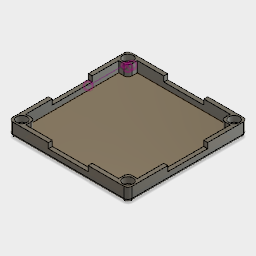
stage0 v2 (Autodesk Fusion 360 design; units mm, degrees)
Autodesk Fusion 360 part; units mm, degrees
sketch "Sketch1" plane through (0, 0, 0) normal (0, 1, 0) x (1, 0, 0)
  line L0 (0, 0) -> (90, 0)
  line L1 (90, 0) -> (90, 90)
  line L2 (90, 90) -> (0, 90)
  line L3 (0, 90) -> (0, 0)
  dimension "d1" = 90
  dimension "d2" = 90
  measures "d1" distance of L0.start L2.end
  measures "d2" distance of L0.start L0.end
extrude "Extrude1" add sketch "Sketch1" along normal blind 11
sketch "Sketch2" plane through (0, 11, 0) normal (0, 1, 0) x (-1, 0, 0)
  line L0 (0, -90) -> (0, 0)
  line L1 (0, 0) -> (-90, 0)
  line L2 (-90, 0) -> (-90, -90)
  line L3 (-90, -90) -> (0, -90)
  circle A0 centre (-5, -85) radius 3.875
  circle A1 centre (-5, -5) radius 3.875
  circle A2 centre (-85, -5) radius 3.875
  circle A3 centre (-85, -85) radius 3.875
  dimension "d5" = 7.75
  dimension "d6" = 7.75
  dimension "d7" = 7.75
  dimension "d8" = 7.75
  measures "d5" diameter of A0
  measures "d6" diameter of A1
  measures "d7" diameter of A2
  measures "d8" diameter of A3
extrude "Extrude2" cut sketch "Sketch2" against normal blind 4.5 contours A0 | A1 | A2 | A3
sketch "Sketch3" plane through (0, 11, 0) normal (0, 1, 0) x (-1, 0, 0)
  circle A0 centre (-85, -85) radius 3.875
  circle A1 centre (-5, -5) radius 3.875
  circle A2 centre (-5, -85) radius 3.875
  circle A3 centre (-85, -5) radius 3.875
  line L0 (0, -90) -> (0, 0)
  line L1 (0, 0) -> (-90, 0)
  line L2 (-90, 0) -> (-90, -90)
  line L3 (-90, -90) -> (0, -90)
  line L4 (-90, -80) -> (-90, -10)
  line L5 (0, -10) -> (0, -80)
  line L6 (-10, -90) -> (-80, -90)
  line L7 (-80, 0) -> (-10, 0)
  line L8 (-10, 0) -> (-10, -7)
  line L9 (-10, -83) -> (-10, -90)
  line L10 (-90, -10) -> (-83, -10)
  line L11 (-7, -10) -> (0, -10)
  line L12 (-80, -90) -> (-80, -83)
  line L13 (-80, -7) -> (-80, 0)
  line L14 (0, -80) -> (-7, -80)
  line L15 (-83, -80) -> (-90, -80)
  line L16 (0, -10) -> (-3, -10)
  line L17 (-3, -10) -> (-3, -30)
  line L18 (-3, -30) -> (0, -30)
  line L19 (0, -30) -> (0, -10)
  line L20 (0, -80) -> (-3, -80)
  line L21 (-3, -80) -> (-3, -60)
  line L22 (-3, -60) -> (0, -60)
  line L23 (0, -60) -> (0, -80)
  line L24 (-10, -90) -> (-30, -90)
  line L25 (-30, -90) -> (-30, -87)
  line L26 (-30, -87) -> (-10, -87)
  line L27 (-10, -87) -> (-10, -90)
  line L28 (-80, -90) -> (-60, -90)
  line L29 (-60, -90) -> (-60, -87)
  line L30 (-60, -87) -> (-80, -87)
  line L31 (-80, -87) -> (-80, -90)
  line L32 (-90, -80) -> (-87, -80)
  line L33 (-87, -80) -> (-87, -60)
  line L34 (-87, -60) -> (-90, -60)
  line L35 (-90, -60) -> (-90, -80)
  line L36 (-90, -10) -> (-87, -10)
  line L37 (-87, -10) -> (-87, -30)
  line L38 (-87, -30) -> (-90, -30)
  line L39 (-90, -30) -> (-90, -10)
  line L40 (-80, 0) -> (-60, 0)
  line L41 (-60, 0) -> (-60, -3)
  line L42 (-60, -3) -> (-80, -3)
  line L43 (-80, -3) -> (-80, 0)
  line L44 (-10, 0) -> (-30, 0)
  line L45 (-30, 0) -> (-30, -3)
  line L46 (-30, -3) -> (-10, -3)
  line L47 (-10, -3) -> (-10, 0)
  arc A4 (-10, -7) -> (-7, -10) centre (-7, -7) ccw
  arc A5 (-83, -10) -> (-80, -7) centre (-83, -7) ccw
  arc A6 (-80, -83) -> (-83, -80) centre (-83, -83) ccw
  arc A7 (-7, -80) -> (-10, -83) centre (-7, -83) ccw
  dimension "d11" = 20
  dimension "d12" = 3
  dimension "d13" = 20
  dimension "d14" = 3
  dimension "d15" = 20
  dimension "d16" = 3
  dimension "d17" = 20
  dimension "d18" = 3
  dimension "d19" = 3
  dimension "d20" = 20
  dimension "d21" = 3
  dimension "d22" = 20
  dimension "d23" = 3
  dimension "d24" = 20
  dimension "d25" = 20
  dimension "d26" = 3
  dimension "d27" = 3
  dimension "d28" = 3
  measures "d11" distance of L5.start L18.end
  measures "d12" distance of L5.start L16.end
  measures "d13" distance of L5.end L22.end
  measures "d14" distance of L5.end L20.end
  measures "d15" distance of L6.start L24.end
  measures "d16" distance of L6.start L26.end
  measures "d17" distance of L6.end L28.end
  measures "d18" distance of L6.end L30.end
  measures "d19" distance of L4.start L32.end
  measures "d20" distance of L4.start L34.end
  measures "d21" distance of L4.end L36.end
  measures "d22" distance of L4.end L38.end
  measures "d23" distance of L7.start L42.end
  measures "d24" distance of L7.start L40.end
  measures "d25" distance of L7.end L44.end
  measures "d26" distance of L7.end L46.end
  measures "d27" radius of A4
  measures "d28" radius of A5
extrude "Extrude3" cut sketch "Sketch3" against normal blind 8 contours L0 L1 L2 L3 L4 L5 L6 L7 L8 L9 L10 L11 L12 L13 L14 L15 L17 L18 L21 L22 L25 L26 L29 L30 L33 L34 L37 L38 L41 L42 L45 L46 A4 A5 A6 A7
sketch "Sketch4" plane through (0, 3, 0) normal (0, 1, 0) x (-1, 0, 0)
  line L0 (-3, -80) -> (-3, -60)
  line L1 (-3, -60) -> (0, -60)
  line L2 (0, -60) -> (0, -30)
  line L3 (0, -30) -> (-3, -30)
  line L4 (-3, -30) -> (-3, -10)
  line L5 (-3, -10) -> (-7, -10)
  arc A0 (-10, -7) -> (-7, -10) centre (-7, -7) ccw
  line L6 (-10, -7) -> (-10, -3)
  line L7 (-10, -3) -> (-30, -3)
  line L8 (-30, -3) -> (-30, 0)
  line L9 (-30, 0) -> (-60, 0)
  line L10 (-60, 0) -> (-60, -3)
  line L11 (-60, -3) -> (-80, -3)
  line L12 (-80, -3) -> (-80, -7)
  arc A1 (-83, -10) -> (-80, -7) centre (-83, -7) ccw
  line L13 (-83, -10) -> (-87, -10)
  line L14 (-87, -10) -> (-87, -30)
  line L15 (-87, -30) -> (-90, -30)
  line L16 (-90, -30) -> (-90, -60)
  line L17 (-90, -60) -> (-87, -60)
  line L18 (-87, -60) -> (-87, -80)
  line L19 (-87, -80) -> (-83, -80)
  arc A2 (-80, -83) -> (-83, -80) centre (-83, -83) ccw
  line L20 (-80, -83) -> (-80, -87)
  line L21 (-80, -87) -> (-60, -87)
  line L22 (-60, -87) -> (-60, -90)
  line L23 (-60, -90) -> (-30, -90)
  line L24 (-30, -90) -> (-30, -87)
  line L25 (-30, -87) -> (-10, -87)
  line L26 (-10, -87) -> (-10, -83)
  arc A3 (-7, -80) -> (-10, -83) centre (-7, -83) ccw
  line L27 (-7, -80) -> (-3, -80)
  line L28 (0, -60) -> (-3, -60)
  line L29 (-3, -60) -> (-3, -30)
  line L30 (-3, -30) -> (0, -30)
  line L31 (0, -30) -> (0, -60)
  line L32 (-87, -30) -> (-90, -30)
  line L33 (-90, -30) -> (-90, -60)
  line L34 (-90, -60) -> (-87, -60)
  line L35 (-87, -60) -> (-87, -30)
  line L36 (-30, 0) -> (-60, 0)
  line L37 (-60, 0) -> (-60, -3)
  line L38 (-60, -3) -> (-30, -3)
  line L39 (-30, -3) -> (-30, 0)
  line L40 (-30, -90) -> (-60, -90)
  line L41 (-60, -90) -> (-60, -87)
  line L42 (-60, -87) -> (-30, -87)
  line L43 (-30, -87) -> (-30, -90)
extrude "Extrude4" add sketch "Sketch4" along normal blind 4 contours L1 L2 L3 L28 L29 L30 L31 | L22 L23 L24 L40 L41 L42 L43 | L8 L9 L10 L36 L37 L38 L39 | L15 L16 L17 L32 L33 L34 L35
fillet "Fillet1" radius 3 8 edges at (90, 5.5, 0) (90, 0, -45) (45, 0, 0) (90, 5.5, -90) (45, 0, -90) (0, 5.5, -90) (0, 0, -45) (0, 5.5, 0)
sketch "Sketch6" plane through (0, 3, 0) normal (0, 1, 0) x (-1, 0, 0)
  line L0 (-87, -10) -> (-87, -80)
  line L1 (-87, -80) -> (-83, -80)
  arc A0 (-80, -83) -> (-83, -80) centre (-83, -83) ccw
  line L2 (-80, -83) -> (-80, -87)
  line L3 (-80, -87) -> (-10, -87)
  line L4 (-10, -87) -> (-10, -83)
  arc A1 (-7, -80) -> (-10, -83) centre (-7, -83) ccw
  line L5 (-7, -80) -> (-3, -80)
  line L6 (-3, -80) -> (-3, -10)
  line L7 (-3, -10) -> (-7, -10)
  arc A2 (-10, -7) -> (-7, -10) centre (-7, -7) ccw
  line L8 (-10, -7) -> (-10, -3)
  line L9 (-10, -3) -> (-80, -3)
  line L10 (-80, -3) -> (-80, -7)
  arc A3 (-83, -10) -> (-80, -7) centre (-83, -7) ccw
  line L11 (-83, -10) -> (-87, -10)
  arc A4 (-3, -90) -> (0, -87) centre (-3, -87) ccw
  line L12 (0, -87) -> (0, -60)
sketch "Sketch7" plane through (45, 3, -45) normal (0, 1, 0) x (-1, 0, 0)
